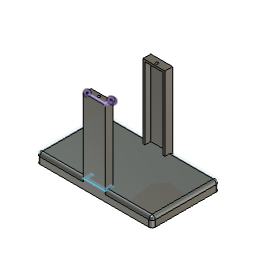
Base (Autodesk Fusion 360 design; units mm, degrees)
Autodesk Fusion 360 part; units mm, degrees
sketch "Sketch1" plane through (0, 0, 0) normal (0, 0, 1) x (1, 0, 0)
  line L0 (0, 0) -> (-180, 0)
  line L1 (-180, 0) -> (-180, 105)
  line L2 (-180, 105) -> (0, 105)
  line L3 (0, 105) -> (0, 0)
  dimension "d1" = 180
  dimension "d2" = 105
  constraint horizontal L0
  constraint vertical L1
  constraint horizontal L2
  constraint vertical L3
  constraint coincident L0.start L3.end
  measures "d1" distance of L0.start L0.end
  measures "d2" distance of L0.start L2.end
extrude "Extrude1" add sketch "Sketch1" along normal blind 15
sketch "Sketch2" plane through (0, 0, 15) normal (0, 0, 1) x (-1, 0, 0)
  line L0 (0, -105) -> (180, -105)
  line L1 (180, -105) -> (180, 0)
  line L2 (180, 0) -> (0, 0)
  line L3 (0, 0) -> (0, -105)
  line L4 (90, 0) -> (73, 0)
  line L5 (90, 0) -> (107, 0)
  line L6 (107, 0) -> (107, -12)
  line L7 (107, -12) -> (104, -12)
  line L8 (104, -12) -> (104, -3)
  line L9 (73, 0) -> (73, -12)
  line L10 (73, -12) -> (76, -12)
  line L11 (76, -12) -> (76, -3)
  line L12 (76, -3) -> (104, -3)
  dimension "d6" = 17
  dimension "d7" = 17
  dimension "d14" = 3
  dimension "d15" = 9
  dimension "d26" = 12
  dimension "d27" = 3
  constraint parallel L2 L4
  constraint parallel L2 L5
  constraint perpendicular L2 L6
  constraint perpendicular L6 L7
  constraint perpendicular L7 L8
  constraint perpendicular L2 L9
  constraint perpendicular L9 L10
  constraint perpendicular L10 L11
  measures "d6" distance of L4.start L4.end
  measures "d7" distance of L4.start L5.end
  measures "d14" distance of L6.end L7.end
  measures "d15" distance of L7.end L8.end
  measures "d26" distance of L4.end L9.end
  measures "d27" distance of L9.end L10.end
extrude "Extrude3" add sketch "Sketch2" along normal blind 115 contours L2 L4 L5 L6 L7 L8 L9 L10 L11 L12
sketch "Sketch4" plane through (0, 0, 130) normal (0, 0, 1) x (-1, 0, 0)
  line L0 (107, 0) -> (73, 0)
  line L1 (104, -3) -> (104, -12)
  line L2 (104, -12) -> (107, -12)
  line L3 (107, -12) -> (107, 0)
  line L4 (73, -12) -> (76, -12)
  line L5 (76, -12) -> (76, -3)
  line L6 (73, 0) -> (73, -12)
  line L7 (76, -3) -> (104, -3)
sketch "Sketch5" plane through (0, 0, 130) normal (0, 0, 1) x (-1, 0, 0)
  line L0 (76, -3) -> (104, -3)
  line L1 (104, -3) -> (104, -12)
  line L2 (104, -12) -> (76, -12)
  line L3 (76, -12) -> (76, -3)
  line L4 (76, -3) -> (104, -12)
  line L5 (76, -12) -> (104, -3)
  circle A0 centre (90, -7.5) radius 2
  dimension "d28" = 4
  constraint horizontal L0
  constraint vertical L1
  constraint horizontal L2
  constraint vertical L3
  constraint midpoint L4 A0.centre
  measures "d28" diameter of A0
extrude "Extrude4" add sketch "Sketch5" against normal blind 3 contours L3 L4 L5 A0 | L0 L4 L5 A0 | L1 L4 L5 A0 | L2 L4 L5 A0
mirror "Mirror2" about plane through (-90, 52.5, 65) normal (0, -1, 0) of "Extrude3", "Extrude4"
ref_plane "WorkPlane3" through (-90, 52.5, 65) normal (0, 1, 0) x (-1, 0, 0)
fillet "Fillet2" radius 5 10 edges at (0, 52.5, 15) (0, 0, 7.5) (0, 105, 7.5) (-180, 52.5, 15) (-180, 105, 7.5) (-180, 0, 7.5) (-143.5, 0, 15) (-143.5, 105, 15) (-36.5, 0, 15) (-36.5, 105, 15)
